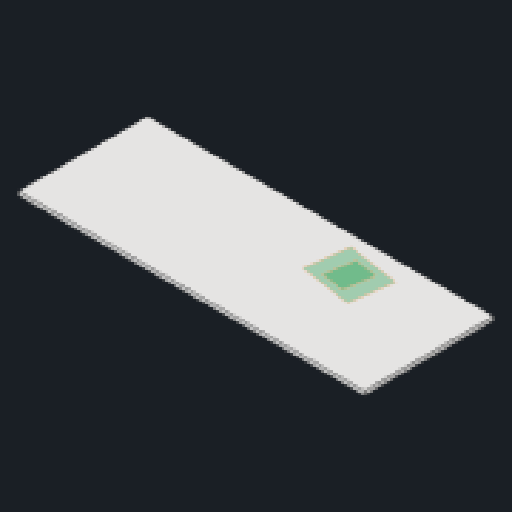
# Autodesk Inventor part: right_gear_holder
Saved by Autodesk Inventor 2023 (Build 270158000, 158)
## iProperties
Created: 2024-04-30
Part Number: right_gear_holder
Material: Generic
Document SubType Name: Modeling
Designer: szymo
Density: 1 g/cm^3
Appearance: Default
Author: szymo
Autodesk Inventor part; units mm, degrees
ref_plane "YZ Plane" through (0, 0, 0) normal (1, 0, 0) x (0, 1, 0)
ref_plane "XZ Plane" through (0, 0, 0) normal (0, 1, 0) x (-1, 0, 0)
ref_plane "XY Plane" through (0, 0, 0) normal (0, 0, 1) x (1, 0, 0)
ref_plane "Work Plane1" through (66, 11, 8.5) normal (0, -1, 0) x (0.1498, 0, -0.9887)
ref_plane "Work Plane2" through (65.6255, 11, 10.9718) normal (0, -1, 0) x (0.1498, 0, -0.9887)
sketch "Sketch2" plane through (65.6255, 11, 10.9718) normal (0, -1, 0) x (0.1498, 0, -0.9887)
  line L0 (-9.1533, -157.0261) -> (10.6197, -26.5155) projected
  line L1 (10.6197, -26.5155) -> (7.1592, -25.9912) projected
  line L2 (-12.6138, -156.5018) -> (7.1592, -25.9912) projected
  line L3 (-9.1533, -157.0261) -> (-12.6138, -156.5018) projected
  line L4 (10.6197, -26.5155) -> (18.1095, 22.9204) projected
  line L5 (18.1095, 22.9204) -> (14.649, 23.4447) projected
  line L6 (7.1592, -25.9912) -> (14.649, 23.4447) projected
  line L7 (10.6197, -26.5155) -> (7.1592, -25.9912) projected
  circle A0 centre (2.9555, -29.9965) radius 2 projected
  line L8 (-27.0486, -51.5049) -> (-11.7235, -53.8267) projected
  line L9 (-27.0486, -51.5049) -> (-15.0125, 27.9385) projected
  line L10 (-27.0486, -51.5049) -> (-15.0125, 27.9385)
  line L11 (-15.0125, 27.9385) -> (14.649, 23.4447)
  line L12 (14.649, 23.4447) -> (2.6129, -55.9987)
  line L13 (-27.0486, -51.5049) -> (2.6129, -55.9987)
  point P0 (1.0176, -66.5286)
  point P1 (-11.7235, -53.8267)
  constraints: 8 end point, 2 perpendicular, 1 collinear, 1 point on line
extrude "Extrusion1" add sketch "Sketch2" along normal blind 1 contours L2 L13 L8 L9 L11 L6 | A0
body "Solid1"
